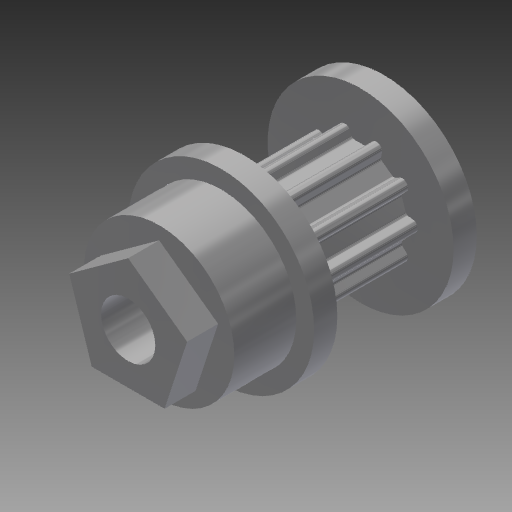
# Autodesk Inventor part: Synchrone Riemenscheibe3
Saved by Autodesk Inventor 2019.1 (Build 231200000, 200)
## iProperties
Created: 2018-11-28
Part Number: Synchrone Riemenscheibe3
Material: Steel
Document SubType Name: Modeling
Designer: JochenAlt
Density: 1 g/cm^3
Appearance: Steel
CustomPartVersion: 1
Author: JochenAlt
Autodesk Inventor part; units mm, degrees
ref_plane "YZ Plane" through (0, 0, 0) normal (1, 0, 0) x (0, 1, 0)
ref_plane "XZ Plane" through (0, 0, 0) normal (0, 1, 0) x (-1, 0, 0)
ref_plane "XY Plane" through (0, 0, 0) normal (0, 0, 1) x (1, 0, 0)
sketch "Riemenscheibenskizze" plane through (0, 0, 0) normal (0, 0, 1) x (1, 0, 0)
  circle A0 centre (0, 0) radius 3.9789 construction
  circle A1 centre (0, 0) radius 3.6789
  circle A2 centre (0, 0) radius 2.9289
  line L0 (-0.8305, 3.5839) -> (-0.525, 2.9289)
  line L1 (-0.525, 2.9289) -> (0.525, 2.9289)
  line L2 (0.525, 2.9289) -> (0.8305, 3.5839)
  line L3 (0, 0) -> (0, 3.6789) construction
  point P0 (0, 2.9289)
  dimension "d0" = 7.9577
  dimension "d1" = 0.3
  dimension "d2" = 0.75
  dimension "d3" = 50
  dimension "d4" = 1.05
  constraints: 8 end point, 3 coincident, 3 point on circle, 2 centre point, 1 horizontal, 1 midpoint, 1 point on line, 1 vertical, 1 vertical alignment, 3 other
  measures "d0" diameter of A0
  measures "d1" radial gap between concentric circles of A0 A1
  measures "d3" angle of L2 L0
  measures "d4" distance of L0.end L1.end
extrude "Grundkörper" add sketch "Riemenscheibenskizze" along normal mid plane 7.5 contours A2 | A1 L0 L1 L2 | L2 L1 L0 A1
extrude "Zahn" cut sketch "Riemenscheibenskizze" along normal through all both and the other way through all contours L2 L1 L0 A1 picked at (0, 3.4218)
fillet "Fillet" radius 0.2 2 edges at (0.525, 2.9289, 0) (-0.525, 2.9289, 0)
fillet "Fillet" radius 0.3 4 edges at (-0.8305, 3.5839, 1.875) (-0.8305, 3.5839, -1.875) (0.8305, 3.5839, 1.875) (0.8305, 3.5839, -1.875)
pattern_circular "Zähne" count 10 over 360 about axis through (0, 0, -10) along (0, 0, 1) of "Zahn", "Fillet"
feature "Flansch links" [suppressed]
feature "Flansch rechts" [suppressed]
sketch "Skizze2" plane through (0, 0, 3.75) normal (0, 0, 1) x (1, 0, 0)
  circle A0 centre (0, 0) radius 4.85
  circle A1 centre (0, 0) radius 1.75
  circle A2 centre (0, 0) radius 6
  circle A3 centre (0, 0) radius 4 construction
  line L0 (0, 4) -> (3.8042, 1.2361)
  line L1 (3.8042, 1.2361) -> (2.3511, -3.2361)
  line L2 (2.3511, -3.2361) -> (-2.3511, -3.2361)
  line L3 (-2.3511, -3.2361) -> (-3.8042, 1.2361)
  line L4 (-3.8042, 1.2361) -> (0, 4)
  dimension "d17" = 9.7
  dimension "d22" = 3.5
  dimension "d27" = 12
  constraints: 10 end point, 5 coincident, 3 centre point, 1 vertical alignment, 13 other
  measures "d17" diameter of A0
  measures "d22" diameter of A1
  measures "d27" diameter of A2
extrude "Extrusion6" add sketch "Skizze2" along normal blind 1.5 contours A0 | A1 | A2 | L0 L1 L2 L3 L4
extrude "Extrusion13" add sketch "Skizze2" along normal blind 4 from surface at 1.5 contours A0 | L0 L1 L2 L3 L4
extrude "Extrusion11" add sketch "Skizze2" along normal blind 2 from surface at 5.5 contours L0 L1 L2 L3 L4
extrude "Extrusion8" add sketch "Skizze2" against normal blind 1.5 from surface at -7.5 contours A0 | A1 | A2 | L0 L1 L2 L3 L4
extrude "Extrusion10" cut sketch "Skizze2" along normal through all both and the other way through all contours A1
extrude "Extrusion12" add sketch "Skizze2" along normal blind 3 contours A0 | A1 | L0 L1 L2 L3 L4
extrude "Extrusion14" cut sketch "Skizze2" along normal through all both and the other way through all contours A1
equation "\"d1\" = da_a"
equation "\"d2\" = da_hg"
equation "\"d3\" = 2 * da_fi"
equation "\"d4\" = da_bw"
equation "\"d5\" = da_bf"
equation "\"d7\" = da_bf"
equation "\"d9\" = da_rb"
equation "\"d10\" = da_rt"
equation "\"da_pb\" = 2.5"
equation "\"da_fi\" = 25deg"
equation "\"da_hg\" = 0.75"
equation "\"da_bw\" = 1.05"
equation "\"da_rb\" = 0.2"
equation "\"da_rt\" = 0.3"
equation "\"da_a\" = 0.3"
equation "\"da_bf\" = 7.5"
equation "\"da_wf\" = 1.5"
equation "\"da_hf\" = 1.5"
body "Solid1"
